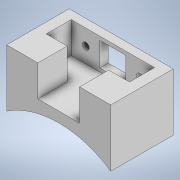
# Autodesk Inventor part: BracketForScope
Saved by Autodesk Inventor 2022.2 (Build 262287000, 287)
## iProperties
Created: 2021-12-26
Part Number: BracketForScope
Material: Generic
Document SubType Name: Modeling
Designer: robst
Density: 1 g/cm^3
Appearance: Default
Author: robst
Autodesk Inventor part; units mm, degrees
note: some values were not read from the file. Chosen so that the rebuilt part matches the saved one: direction of "Hole1".
ref_plane "YZ Plane" through (0, 0, 0) normal (1, 0, 0) x (0, 1, 0)
ref_plane "XZ Plane" through (0, 0, 0) normal (0, 1, 0) x (-1, 0, 0)
sketch "Sketch1" plane through (0, 0, 0) normal (0, 0, 1) x (1, 0, 0)
  arc A0 (25, 37.4166) -> (-25, 37.4166) centre (0, 0) ccw
  line L0 (0, 0) -> (0, 45) construction
  line L1 (0, 45) -> (25, 45)
  line L2 (0, 45) -> (-25, 45)
  line L3 (-25, 45) -> (-25, 37.4166)
  line L4 (25, 45) -> (25, 37.4166)
  line L5 (-25, 45) -> (25, 45)
  line L6 (25, 45) -> (25, 50)
  line L7 (25, 50) -> (-25, 50)
  line L8 (-25, 50) -> (-25, 45)
  dimension "d0" = 90
  dimension "d1" = 50
  dimension "d2" = 5
  constraints: 18 end point, 3 horizontal, 3 parallel, 3 point on circle, 2 vertical, 1 centre point, 1 coincident, 1 collinear, 1 perpendicular, 1 tangent
  measures "d0" diameter of A0
  measures "d1" distance of L1.end L2.end
  measures "d2" distance of L7.end L2.end
extrude "Extrusion1" add sketch "Sketch1" along normal mid plane 30
sketch "Sketch2" plane through (-25, 50, 15) normal (0, 1, 0) x (1, 0, 0)
  line L0 (50, 0) -> (0, 0) construction
  line L1 (25, 0) -> (25, 29.8898) construction
  line L2 (50, 0) -> (0, 0) construction
  line L3 (15, 0) -> (35, 0)
  line L4 (35, 0) -> (35, 14)
  line L5 (35, 14) -> (15, 14)
  line L6 (15, 14) -> (15, 0)
  line L7 (15, 0) -> (35, 14) construction
  line L8 (35, 0) -> (15, 14) construction
  line L9 (5, 14) -> (45, 14)
  line L10 (45, 14) -> (45, 26)
  line L11 (45, 26) -> (5, 26)
  line L12 (5, 26) -> (5, 14)
  line L13 (5, 14) -> (45, 26) construction
  line L14 (45, 14) -> (5, 26) construction
  line L15 (0, 30) -> (50, 30) projected
  line L16 (50, 30) -> (50, 0) projected
  line L17 (0, 0) -> (50, 0)
  line L18 (50, 0) -> (50, 30)
  line L19 (50, 30) -> (0, 30)
  line L20 (0, 30) -> (0, 0)
  point P0 (25, 15)
  point P1 (25, 7)
  point P2 (25, 20)
  point P3 (35, 14)
  point P4 (35, 0)
  point P5 (15, 0)
  point P6 (15, 14)
  dimension "d5" = 20
  dimension "d6" = 14
  dimension "d7" = 40
  dimension "d8" = 12
  dimension "d9" = 4
  dimension "d24" = 50
  constraints: 34 end point, 6 parallel, 5 midpoint, 5 perpendicular, 2 collinear, 2 point on line, 1 horizontal, 1 vertical
  measures "d5" distance of L4.end L5.end
  measures "d6" distance of L5.end L3.start
  measures "d7" distance of L10.end L11.end
  measures "d8" distance of L11.end L9.start
  measures "d9" distance between parallel lines of L11 L15
  measures "d24" distance between parallel lines of L18 L20
extrude "Extrusion2" add sketch "Sketch2" along normal blind 15 contours L17 L20 L15 L16 L4 L9 L10 L11 L12 L6
sketch "Sketch3" plane through (0, 0, -15) normal (0, 0, -1) x (-1, 0, 0)
  line L0 (-20, 50) -> (20, 50) projected
  line L1 (-25, 65) -> (25, 65) projected
  line L2 (20, 50) -> (20, 65) projected
  line L3 (-20, 50) -> (-20, 65) projected
  line L4 (0, 65) -> (0, 50) construction
  line L5 (20, 50) -> (20, 65) construction
  line L6 (20, 57.5) -> (-20, 57.5) construction
  line L7 (-6.25, 63.25) -> (-6.25, 51.75)
  line L8 (-6.25, 51.75) -> (6.25, 51.75)
  line L9 (6.25, 51.75) -> (6.25, 63.25)
  line L10 (6.25, 63.25) -> (-6.25, 63.25)
  line L11 (-6.25, 63.25) -> (6.25, 51.75) construction
  line L12 (-6.25, 51.75) -> (6.25, 63.25) construction
  point P0 (0, 0)
  point P1 (0, 57.5)
  dimension "d12" = 11.5
  dimension "d13" = 12.5
  constraints: 16 end point, 7 midpoint, 2 parallel, 1 perpendicular, 1 vertical
  measures "d12" distance of L8.end L9.end
  measures "d13" distance of L9.end L7.start
extrude "Extrusion3" cut sketch "Sketch3" against normal up to surface (4 mm away) contours L10 L9 L8 L7
sketch "Sketch5" plane through (0, 0, -15) normal (0, 0, -1) x (-1, 0, 0)
  line L0 (-20, 50) -> (20, 50) projected
  line L1 (20, 50) -> (20, 65) projected
  line L2 (-20, 50) -> (-20, 65) projected
  line L3 (-10, 50) -> (10, 50) construction
  line L4 (0, 50) -> (0, 65) construction
  line L5 (0, 57.5) -> (13, 57.5) construction
  line L6 (0, 57.5) -> (-13, 57.5) construction
  line L7 (6.25, 63.25) -> (6.25, 51.75) projected
  line L8 (-6.25, 51.75) -> (-6.25, 63.25) projected
  line L9 (6.25, 51.75) -> (6.25, 63.25) construction
  line L10 (6.25, 57.5) -> (-6.25, 57.5) construction
  line L11 (-6.25, 63.25) -> (-6.25, 51.75) construction
  point P0 (0, 0)
  dimension "d16" = 26
  constraints: 8 end point, 4 midpoint, 2 coincident, 2 collinear, 2 horizontal, 1 vertical
  measures "d16" distance of L5.end L6.end
hole "Hole1" at (13, 57.5, -15) at (-13, 57.5, -15) direction (0, 0, 1) diameter 3.264 end up to surface clearance for "Flat Head Machine Screw (82)" size "#4" standard "Ansi Unified Screw Threads"
ref_plane "Work Plane2" through (25, 37.4166, 0) normal (0, -1, 0) x (0, 0, 1)
sketch "Sketch6" plane through (25, 37.4166, 0) normal (0, -1, 0) x (0, 0, 1)
  line L0 (-15, 0) -> (-15, 50) projected
  line L1 (15, 50) -> (15, 0) projected
  line L2 (-15, 0) -> (15, 0) projected
  line L3 (-15, 50) -> (15, 50) projected
  line L4 (15, 0) -> (-15, 0) construction
  line L5 (0, 0) -> (0, 50) construction
  spline S0 degree 2 poles (0.1264, 5.3857) (0.1264, 4.8558) (-0.1507, 4.0681) (-0.4279, 3.7909) knots 0 0 0 1 2 2 2
  spline S1 degree 2 poles (-0.4279, 3.7909) (-0.7391, 3.4749) (-1.6143, 3.2172) (-2.2561, 3.2172) knots 0 0 0 1 2 2 2
  line L6 (-2.2561, 3.2172) -> (-6, 3.2172)
  line L7 (-6, 3.2172) -> (-6, 4.0146)
  line L8 (-6, 4.0146) -> (-2.2561, 4.0146)
  spline S2 degree 2 poles (-2.2561, 4.0146) (-1.8379, 4.0146) (-1.2739, 4.1216) (-1.0454, 4.2723) knots 0 0 0 1 2 2 2
  spline S3 degree 2 poles (-1.0454, 4.2723) (-0.8023, 4.4327) (-0.5543, 4.987) (-0.5543, 5.3857) knots 0 0 0 1 2 2 2
  spline S4 degree 2 poles (-0.5543, 5.3857) (-0.5543, 5.7601) (-0.8023, 6.3436) (-1.0454, 6.5041) knots 0 0 0 1 2 2 2
  spline S5 degree 2 poles (-1.0454, 6.5041) (-1.2739, 6.6548) (-1.8331, 6.7617) (-2.2366, 6.7617) knots 0 0 0 1 2 2 2
  line L9 (-2.2366, 6.7617) -> (-6, 6.7617)
  line L10 (-6, 6.7617) -> (-6, 7.5592)
  line L11 (-6, 7.5592) -> (-2.2561, 7.5592)
  spline S6 degree 2 poles (-2.2561, 7.5592) (-1.6288, 7.5592) (-0.7342, 7.3063) (-0.4279, 6.9854) knots 0 0 0 1 2 2 2
  spline S7 degree 2 poles (-0.4279, 6.9854) (-0.1459, 6.6985) (0.1264, 5.94) (0.1264, 5.3857) knots 0 0 0 1 2 2 2
  spline S8 degree 2 poles (0.107, 10.3744) (0.107, 9.7229) (-0.1653, 8.8088) (-0.3598, 8.4052) knots 0 0 0 1 2 2 2
  line L12 (-0.3598, 8.4052) -> (-1.3614, 8.4052)
  line L13 (-1.3614, 8.4052) -> (-1.3614, 8.4635)
  spline S9 degree 2 poles (-1.3614, 8.4635) (-0.9919, 8.8574) (-0.5835, 9.8541) (-0.5835, 10.316) knots 0 0 0 1 2 2 2
  spline S10 degree 2 poles (-0.5835, 10.316) (-0.5835, 10.9773) (-1.1329, 11.6532) (-1.5851, 11.6532) knots 0 0 0 1 2 2 2
  spline S11 degree 2 poles (-1.5851, 11.6532) (-1.9449, 11.6532) (-2.3922, 11.2982) (-2.5041, 10.9141) knots 0 0 0 1 2 2 2
  spline S12 degree 2 poles (-2.5041, 10.9141) (-2.5818, 10.637) (-2.6888, 10.175) (-2.7763, 9.8298) knots 0 0 0 1 2 2 2
  spline S13 degree 2 poles (-2.7763, 9.8298) (-2.859, 9.5186) (-3.107, 9.0276) (-3.3063, 8.8379) knots 0 0 0 1 2 2 2
  spline S14 degree 2 poles (-3.3063, 8.8379) (-3.5057, 8.6532) (-4.0405, 8.4489) (-4.3906, 8.4489) knots 0 0 0 1 2 2 2
  spline S15 degree 2 poles (-4.3906, 8.4489) (-5.1199, 8.4489) (-6.107, 9.5867) (-6.107, 10.4668) knots 0 0 0 1 2 2 2
  spline S16 degree 2 poles (-6.107, 10.4668) (-6.107, 10.9724) (-5.9076, 11.8671) (-5.718, 12.2512) knots 0 0 0 1 2 2 2
  line L14 (-5.718, 12.2512) -> (-4.765, 12.2512)
  line L15 (-4.765, 12.2512) -> (-4.765, 12.1929)
  spline S17 degree 2 poles (-4.765, 12.1929) (-5.0276, 11.906) (-5.4165, 11.0113) (-5.4165, 10.5203) knots 0 0 0 1 2 2 2
  spline S18 degree 2 poles (-5.4165, 10.5203) (-5.4165, 9.966) (-4.8963, 9.2804) (-4.4733, 9.2804) knots 0 0 0 1 2 2 2
  spline S19 degree 2 poles (-4.4733, 9.2804) (-4.094, 9.2804) (-3.6418, 9.684) (-3.5397, 10.0632) knots 0 0 0 1 2 2 2
  spline S20 degree 2 poles (-3.5397, 10.0632) (-3.4716, 10.316) (-3.2966, 11.0502) (-3.2237, 11.2934) knots 0 0 0 1 2 2 2
  spline S21 degree 2 poles (-3.2237, 11.2934) (-3.034, 11.9109) (-2.2707, 12.4846) (-1.7115, 12.4846) knots 0 0 0 1 2 2 2
  spline S22 degree 2 poles (-1.7115, 12.4846) (-1.3566, 12.4846) (-0.6759, 12.1977) (-0.4376, 11.94) knots 0 0 0 1 2 2 2
  spline S23 degree 2 poles (-0.4376, 11.94) (-0.175, 11.6532) (0.107, 10.9238) (0.107, 10.3744) knots 0 0 0 1 2 2 2
  spline S24 degree 2 poles (-1.8428, 17.3663) (-1.3955, 17.3663) (-0.7099, 17.0259) (-0.4862, 16.7439) knots 0 0 0 1 2 2 2
  spline S25 degree 2 poles (-0.4862, 16.7439) (-0.2237, 16.4036) (0, 15.6305) (0, 15.0178) knots 0 0 0 1 2 2 2
  line L16 (0, 15.0178) -> (0, 13.2966)
  line L17 (0, 13.2966) -> (-6, 13.2966)
  line L18 (-6, 13.2966) -> (-6, 14.8865)
  spline S26 degree 2 poles (-6, 14.8865) (-6, 15.5284) (-5.9173, 16.1702) (-5.7569, 16.4619) knots 0 0 0 1 2 2 2
  spline S27 degree 2 poles (-5.7569, 16.4619) (-5.5867, 16.7877) (-5.0276, 17.0843) (-4.6483, 17.0843) knots 0 0 0 1 2 2 2
  spline S28 degree 2 poles (-4.6483, 17.0843) (-4.2253, 17.0843) (-3.5543, 16.637) (-3.3647, 16.2431) knots 0 0 0 1 2 2 2
  line L19 (-3.3647, 16.2431) -> (-3.3355, 16.2431)
  spline S29 degree 2 poles (-3.3355, 16.2431) (-3.1896, 16.778) (-2.4165, 17.3663) (-1.8428, 17.3663) knots 0 0 0 1 2 2 2
  spline S30 degree 2 poles (-1.8088, 16.5348) (-2.1491, 16.5348) (-2.5867, 16.3404) (-2.7423, 16.0486) knots 0 0 0 1 2 2 2
  spline S31 degree 2 poles (-2.7423, 16.0486) (-2.8395, 15.859) (-2.8979, 15.4117) (-2.8979, 14.9984) knots 0 0 0 1 2 2 2
  line L20 (-2.8979, 14.9984) -> (-2.8979, 14.094)
  line L21 (-2.8979, 14.094) -> (-0.6807, 14.094)
  line L22 (-0.6807, 14.094) -> (-0.6807, 14.7407)
  spline S32 degree 2 poles (-0.6807, 14.7407) (-0.6807, 15.2658) (-0.778, 15.8687) (-0.9335, 16.1021) knots 0 0 0 1 2 2 2
  spline S33 degree 2 poles (-0.9335, 16.1021) (-1.094, 16.3258) (-1.4927, 16.5348) (-1.8088, 16.5348) knots 0 0 0 1 2 2 2
  spline S34 degree 2 poles (-4.5365, 16.2528) (-4.7504, 16.2528) (-5.0713, 16.107) (-5.1637, 15.9465) knots 0 0 0 1 2 2 2
  spline S35 degree 2 poles (-5.1637, 15.9465) (-5.2707, 15.752) (-5.3193, 15.2804) (-5.3193, 14.8574) knots 0 0 0 1 2 2 2
  line L23 (-5.3193, 14.8574) -> (-5.3193, 14.094)
  line L24 (-5.3193, 14.094) -> (-3.564, 14.094)
  line L25 (-3.564, 14.094) -> (-3.564, 14.9984)
  spline S36 degree 2 poles (-3.564, 14.9984) (-3.564, 15.3728) (-3.6418, 15.7277) (-3.7634, 15.9173) knots 0 0 0 1 2 2 2
  spline S37 degree 2 poles (-3.7634, 15.9173) (-3.8801, 16.1021) (-4.2545, 16.2528) (-4.5365, 16.2528) knots 0 0 0 1 2 2 2
  spline S38 degree 2 poles (-1.8428, 24.8055) (-1.3955, 24.8055) (-0.7099, 24.4652) (-0.4862, 24.1831) knots 0 0 0 1 2 2 2
  spline S39 degree 2 poles (-0.4862, 24.1831) (-0.2237, 23.8428) (0, 23.0697) (0, 22.4571) knots 0 0 0 1 2 2 2
  line L26 (0, 22.4571) -> (0, 20.7358)
  line L27 (0, 20.7358) -> (-6, 20.7358)
  line L28 (-6, 20.7358) -> (-6, 22.3258)
  spline S40 degree 2 poles (-6, 22.3258) (-6, 22.9676) (-5.9173, 23.6094) (-5.7569, 23.9011) knots 0 0 0 1 2 2 2
  spline S41 degree 2 poles (-5.7569, 23.9011) (-5.5867, 24.2269) (-5.0276, 24.5235) (-4.6483, 24.5235) knots 0 0 0 1 2 2 2
  spline S42 degree 2 poles (-4.6483, 24.5235) (-4.2253, 24.5235) (-3.5543, 24.0762) (-3.3647, 23.6823) knots 0 0 0 1 2 2 2
  line L29 (-3.3647, 23.6823) -> (-3.3355, 23.6823)
  spline S43 degree 2 poles (-3.3355, 23.6823) (-3.1896, 24.2172) (-2.4165, 24.8055) (-1.8428, 24.8055) knots 0 0 0 1 2 2 2
  spline S44 degree 2 poles (-1.8088, 23.9741) (-2.1491, 23.9741) (-2.5867, 23.7796) (-2.7423, 23.4878) knots 0 0 0 1 2 2 2
  spline S45 degree 2 poles (-2.7423, 23.4878) (-2.8395, 23.2982) (-2.8979, 22.8509) (-2.8979, 22.4376) knots 0 0 0 1 2 2 2
  line L30 (-2.8979, 22.4376) -> (-2.8979, 21.5332)
  line L31 (-2.8979, 21.5332) -> (-0.6807, 21.5332)
  line L32 (-0.6807, 21.5332) -> (-0.6807, 22.1799)
  spline S46 degree 2 poles (-0.6807, 22.1799) (-0.6807, 22.705) (-0.778, 23.3079) (-0.9335, 23.5413) knots 0 0 0 1 2 2 2
  spline S47 degree 2 poles (-0.9335, 23.5413) (-1.094, 23.765) (-1.4927, 23.9741) (-1.8088, 23.9741) knots 0 0 0 1 2 2 2
  spline S48 degree 2 poles (-4.5365, 23.6921) (-4.7504, 23.6921) (-5.0713, 23.5462) (-5.1637, 23.3857) knots 0 0 0 1 2 2 2
  spline S49 degree 2 poles (-5.1637, 23.3857) (-5.2707, 23.1912) (-5.3193, 22.7196) (-5.3193, 22.2966) knots 0 0 0 1 2 2 2
  line L33 (-5.3193, 22.2966) -> (-5.3193, 21.5332)
  line L34 (-5.3193, 21.5332) -> (-3.564, 21.5332)
  line L35 (-3.564, 21.5332) -> (-3.564, 22.4376)
  spline S50 degree 2 poles (-3.564, 22.4376) (-3.564, 22.812) (-3.6418, 23.1669) (-3.7634, 23.3566) knots 0 0 0 1 2 2 2
  spline S51 degree 2 poles (-3.7634, 23.3566) (-3.8801, 23.5413) (-4.2545, 23.6921) (-4.5365, 23.6921) knots 0 0 0 1 2 2 2
  line L36 (-3.6904, 27.9271) -> (-3.6904, 27.8882)
  spline S52 degree 2 poles (-3.6904, 27.8882) (-3.7147, 27.8006) (-3.7245, 27.611) (-3.7245, 27.4797) knots 0 0 0 1 2 2 2
  spline S53 degree 2 poles (-3.7245, 27.4797) (-3.7245, 27.1734) (-3.4571, 26.5705) (-3.1945, 26.2982) knots 0 0 0 1 2 2 2
  line L37 (-3.1945, 26.2982) -> (0, 26.2982)
  line L38 (0, 26.2982) -> (0, 25.5397)
  line L39 (0, 25.5397) -> (-4.5024, 25.5397)
  line L40 (-4.5024, 25.5397) -> (-4.5024, 26.2982)
  line L41 (-4.5024, 26.2982) -> (-3.8314, 26.2982)
  spline S54 degree 2 poles (-3.8314, 26.2982) (-4.201, 26.7115) (-4.5024, 27.329) (-4.5024, 27.6207) knots 0 0 0 1 2 2 2
  spline S55 degree 2 poles (-4.5024, 27.6207) (-4.5024, 27.7374) (-4.4927, 27.8541) (-4.4781, 27.9271) knots 0 0 0 1 2 2 2
  line L42 (-4.4781, 27.9271) -> (-3.6904, 27.9271)
  spline S56 degree 2 poles (-0.4765, 31.0243) (-0.4084, 30.9319) (-0.1653, 30.6207) (-0.0924, 30.4749) knots 0 0 0 1 2 2 2
  spline S57 degree 2 poles (-0.0924, 30.4749) (0.0146, 30.2755) (0.1264, 29.9011) (0.1264, 29.5608) knots 0 0 0 1 2 2 2
  spline S58 degree 2 poles (0.1264, 29.5608) (0.1264, 29.2836) (-0.0827, 28.7828) (-0.2723, 28.5932) knots 0 0 0 1 2 2 2
  spline S59 degree 2 poles (-0.2723, 28.5932) (-0.4571, 28.4133) (-1.0016, 28.1945) (-1.3031, 28.1945) knots 0 0 0 1 2 2 2
  spline S60 degree 2 poles (-1.3031, 28.1945) (-1.7699, 28.1945) (-2.4311, 28.5883) (-2.6207, 29.0162) knots 0 0 0 1 2 2 2
  spline S61 degree 2 poles (-2.6207, 29.0162) (-2.7958, 29.3955) (-2.9271, 30.4263) (-2.9611, 31.0243) knots 0 0 0 1 2 2 2
  line L43 (-2.9611, 31.0243) -> (-3.107, 31.0243)
  spline S62 degree 2 poles (-3.107, 31.0243) (-3.3695, 31.0243) (-3.6953, 30.8639) (-3.7877, 30.718) knots 0 0 0 1 2 2 2
  spline S63 degree 2 poles (-3.7877, 30.718) (-3.8801, 30.5721) (-3.9384, 30.154) (-3.9384, 29.9303) knots 0 0 0 1 2 2 2
  spline S64 degree 2 poles (-3.9384, 29.9303) (-3.9384, 29.6677) (-3.7828, 28.9579) (-3.6321, 28.6029) knots 0 0 0 1 2 2 2
  line L44 (-3.6321, 28.6029) -> (-3.6321, 28.5592)
  line L45 (-3.6321, 28.5592) -> (-4.4052, 28.5592)
  spline S65 degree 2 poles (-4.4052, 28.5592) (-4.4635, 28.7682) (-4.6094, 29.5511) (-4.6094, 29.9352) knots 0 0 0 1 2 2 2
  spline S66 degree 2 poles (-4.6094, 29.9352) (-4.6094, 30.4019) (-4.4635, 31.0389) (-4.2739, 31.2917) knots 0 0 0 1 2 2 2
  spline S67 degree 2 poles (-4.2739, 31.2917) (-4.0891, 31.5397) (-3.5008, 31.7828) (-3.0778, 31.7828) knots 0 0 0 1 2 2 2
  line L46 (-3.0778, 31.7828) -> (0, 31.7828)
  line L47 (0, 31.7828) -> (0, 31.0243)
  line L48 (0, 31.0243) -> (-0.4765, 31.0243)
  line L49 (-1.1086, 31.0243) -> (-2.3582, 31.0243)
  spline S68 degree 2 poles (-2.3582, 31.0243) (-2.3339, 30.752) (-2.2512, 29.9303) (-2.1734, 29.6726) knots 0 0 0 1 2 2 2
  spline S69 degree 2 poles (-2.1734, 29.6726) (-2.081, 29.3712) (-1.6969, 28.9773) (-1.3566, 28.9773) knots 0 0 0 1 2 2 2
  spline S70 degree 2 poles (-1.3566, 28.9773) (-0.9676, 28.9773) (-0.5737, 29.4149) (-0.5737, 29.8331) knots 0 0 0 1 2 2 2
  spline S71 degree 2 poles (-0.5737, 29.8331) (-0.5737, 30.188) (-0.8801, 30.7715) (-1.1086, 31.0243) knots 0 0 0 1 2 2 2
  spline S72 degree 2 poles (0.1021, 34.637) (0.1021, 34.1702) (-0.1848, 33.3971) (-0.4765, 33.1199) knots 0 0 0 1 2 2 2
  spline S73 degree 2 poles (-0.4765, 33.1199) (-0.7634, 32.8428) (-1.6483, 32.5365) (-2.2415, 32.5365) knots 0 0 0 1 2 2 2
  spline S74 degree 2 poles (-2.2415, 32.5365) (-2.8347, 32.5365) (-3.7002, 32.8525) (-3.9919, 33.1199) knots 0 0 0 1 2 2 2
  spline S75 degree 2 poles (-3.9919, 33.1199) (-4.2885, 33.3874) (-4.6045, 34.1799) (-4.6045, 34.637) knots 0 0 0 1 2 2 2
  spline S76 degree 2 poles (-4.6045, 34.637) (-4.6045, 35.0065) (-4.3955, 35.6969) (-4.2593, 35.9643) knots 0 0 0 1 2 2 2
  line L50 (-4.2593, 35.9643) -> (-3.4084, 35.9643)
  line L51 (-3.4084, 35.9643) -> (-3.4084, 35.9206)
  spline S77 degree 2 poles (-3.4084, 35.9206) (-3.4765, 35.8379) (-3.6515, 35.5851) (-3.7439, 35.4052) knots 0 0 0 1 2 2 2
  spline S78 degree 2 poles (-3.7439, 35.4052) (-3.8217, 35.2447) (-3.9433, 34.8169) (-3.9433, 34.6224) knots 0 0 0 1 2 2 2
  spline S79 degree 2 poles (-3.9433, 34.6224) (-3.9433, 34.034) (-3.0535, 33.3193) (-2.2415, 33.3193) knots 0 0 0 1 2 2 2
  spline S80 degree 2 poles (-2.2415, 33.3193) (-1.4489, 33.3193) (-0.5592, 34.0097) (-0.5592, 34.6224) knots 0 0 0 1 2 2 2
  spline S81 degree 2 poles (-0.5592, 34.6224) (-0.5592, 34.9919) (-0.8655, 35.6629) (-1.1037, 35.9206) knots 0 0 0 1 2 2 2
  line L52 (-1.1037, 35.9206) -> (-1.1037, 35.9643)
  line L53 (-1.1037, 35.9643) -> (-0.2528, 35.9643)
  spline S82 degree 2 poles (-0.2528, 35.9643) (-0.1994, 35.8525) (-0.0486, 35.5122) (-0.0146, 35.376) knots 0 0 0 1 2 2 2
  spline S83 degree 2 poles (-0.0146, 35.376) (0.0438, 35.1815) (0.1021, 34.8752) (0.1021, 34.637) knots 0 0 0 1 2 2 2
  line L54 (0, 40.3841) -> (0, 39.3874)
  line L55 (0, 39.3874) -> (-2.1734, 37.7148)
  line L56 (-2.1734, 37.7148) -> (-1.8817, 37.4133)
  line L57 (-1.8817, 37.4133) -> (0, 37.4133)
  line L58 (0, 37.4133) -> (0, 36.6548)
  line L59 (0, 36.6548) -> (-6.2674, 36.6548)
  line L60 (-6.2674, 36.6548) -> (-6.2674, 37.4133)
  line L61 (-6.2674, 37.4133) -> (-2.6013, 37.4133)
  line L62 (-2.6013, 37.4133) -> (-4.5024, 39.1929)
  line L63 (-4.5024, 39.1929) -> (-4.5024, 40.1361)
  line L64 (-4.5024, 40.1361) -> (-2.6207, 38.2885)
  line L65 (-2.6207, 38.2885) -> (0, 40.3841)
  spline S84 degree 2 poles (0.1021, 42.718) (0.1021, 41.6386) (-1.1086, 40.4522) (-2.2269, 40.4522) knots 0 0 0 1 2 2 2
  spline S85 degree 2 poles (-2.2269, 40.4522) (-3.3258, 40.4522) (-4.6288, 41.6045) (-4.6288, 42.5332) knots 0 0 0 1 2 2 2
  spline S86 degree 2 poles (-4.6288, 42.5332) (-4.6288, 42.9514) (-4.3857, 43.5981) (-4.128, 43.8363) knots 0 0 0 1 2 2 2
  spline S87 degree 2 poles (-4.128, 43.8363) (-3.8703, 44.0794) (-3.1264, 44.3371) (-2.5867, 44.3371) knots 0 0 0 1 2 2 2
  line L66 (-2.5867, 44.3371) -> (-2.1734, 44.3371)
  line L67 (-2.1734, 44.3371) -> (-2.1734, 41.2204)
  spline S88 degree 2 poles (-2.1734, 41.2204) (-1.3906, 41.2204) (-0.5592, 42.0081) (-0.5592, 42.7083) knots 0 0 0 1 2 2 2
  spline S89 degree 2 poles (-0.5592, 42.7083) (-0.5592, 42.9562) (-0.671, 43.4376) (-0.7585, 43.6321) knots 0 0 0 1 2 2 2
  spline S90 degree 2 poles (-0.7585, 43.6321) (-0.8558, 43.8363) (-1.0259, 44.1183) (-1.1037, 44.2107) knots 0 0 0 1 2 2 2
  line L68 (-1.1037, 44.2107) -> (-1.1037, 44.2545)
  line L69 (-1.1037, 44.2545) -> (-0.2771, 44.2545)
  spline S91 degree 2 poles (-0.2771, 44.2545) (-0.2237, 44.1232) (-0.0681, 43.7245) (-0.0243, 43.5689) knots 0 0 0 1 2 2 2
  spline S92 degree 2 poles (-0.0243, 43.5689) (0.0389, 43.3501) (0.1021, 42.9903) (0.1021, 42.718) knots 0 0 0 1 2 2 2
  spline S93 degree 2 poles (-2.752, 43.5981) (-3.0583, 43.5883) (-3.5057, 43.4619) (-3.6564, 43.3404) knots 0 0 0 1 2 2 2
  spline S94 degree 2 poles (-3.6564, 43.3404) (-3.8266, 43.2091) (-4.0065, 42.7958) (-4.0065, 42.4895) knots 0 0 0 1 2 2 2
  spline S95 degree 2 poles (-4.0065, 42.4895) (-4.0065, 42.188) (-3.8266, 41.765) (-3.6515, 41.59) knots 0 0 0 1 2 2 2
  spline S96 degree 2 poles (-3.6515, 41.59) (-3.4716, 41.4198) (-3.0389, 41.2447) (-2.752, 41.2204) knots 0 0 0 1 2 2 2
  line L70 (-2.752, 41.2204) -> (-2.752, 43.5981)
  spline S97 degree 2 poles (0.0875, 46.4668) (0.0875, 45.8493) (-0.6175, 45.154) (-1.3809, 45.154) knots 0 0 0 1 2 2 2
  line L71 (-1.3809, 45.154) -> (-3.8752, 45.154)
  line L72 (-3.8752, 45.154) -> (-3.8752, 44.6434)
  line L73 (-3.8752, 44.6434) -> (-4.5024, 44.6434)
  line L74 (-4.5024, 44.6434) -> (-4.5024, 45.154)
  line L75 (-4.5024, 45.154) -> (-5.7958, 45.154)
  line L76 (-5.7958, 45.154) -> (-5.7958, 45.9125)
  line L77 (-5.7958, 45.9125) -> (-4.5024, 45.9125)
  line L78 (-4.5024, 45.9125) -> (-4.5024, 47.3079)
  line L79 (-4.5024, 47.3079) -> (-3.8752, 47.3079)
  line L80 (-3.8752, 47.3079) -> (-3.8752, 45.9125)
  line L81 (-3.8752, 45.9125) -> (-1.731, 45.9125)
  spline S98 degree 2 poles (-1.731, 45.9125) (-1.3906, 45.9125) (-1.0162, 45.9368) (-0.8558, 46.0195) knots 0 0 0 1 2 2 2
  spline S99 degree 2 poles (-0.8558, 46.0195) (-0.7147, 46.0875) (-0.5737, 46.3938) (-0.5737, 46.6564) knots 0 0 0 1 2 2 2
  spline S100 degree 2 poles (-0.5737, 46.6564) (-0.5737, 46.8412) (-0.6856, 47.1864) (-0.7196, 47.2642) knots 0 0 0 1 2 2 2
  line L82 (-0.7196, 47.2642) -> (-0.7196, 47.3079)
  line L83 (-0.7196, 47.3079) -> (-0.0389, 47.3079)
  spline S101 degree 2 poles (-0.0389, 47.3079) (0.0194, 47.094) (0.0875, 46.6564) (0.0875, 46.4668) knots 0 0 0 1 2 2 2
  spline S102 degree 2 poles (5.7169, 20.1596) (6.1059, 20.1596) (6.806, 19.8825) (7.0492, 19.6345) knots 0 0 0 1 2 2 2
  spline S103 degree 2 poles (7.0492, 19.6345) (7.3555, 19.3233) (7.6715, 18.4822) (7.6715, 17.8404) knots 0 0 0 1 2 2 2
  line L84 (7.6715, 17.8404) -> (7.6715, 17.1645)
  line L85 (7.6715, 17.1645) -> (9.9082, 17.1645)
  line L86 (9.9082, 17.1645) -> (9.9082, 16.3671)
  line L87 (9.9082, 16.3671) -> (3.9082, 16.3671)
  line L88 (3.9082, 16.3671) -> (3.9082, 17.8744)
  spline S104 degree 2 poles (3.9082, 17.8744) (3.9082, 18.4092) (4.0832, 19.158) (4.2825, 19.4449) knots 0 0 0 1 2 2 2
  spline S105 degree 2 poles (4.2825, 19.4449) (4.5111, 19.7804) (5.2161, 20.1596) (5.7169, 20.1596) knots 0 0 0 1 2 2 2
  spline S106 degree 2 poles (5.7412, 19.3282) (5.43, 19.3282) (4.973, 19.1143) (4.8271, 18.8955) knots 0 0 0 1 2 2 2
  spline S107 degree 2 poles (4.8271, 18.8955) (4.7007, 18.7058) (4.5986, 18.2002) (4.5986, 17.8258) knots 0 0 0 1 2 2 2
  line L89 (4.5986, 17.8258) -> (4.5986, 17.1645)
  line L90 (4.5986, 17.1645) -> (6.9908, 17.1645)
  line L91 (6.9908, 17.1645) -> (6.9908, 17.7091)
  spline S108 degree 2 poles (6.9908, 17.7091) (6.9908, 18.1953) (6.8352, 18.7934) (6.631, 18.9878) knots 0 0 0 1 2 2 2
  spline S109 degree 2 poles (6.631, 18.9878) (6.4511, 19.1677) (6.0281, 19.3282) (5.7412, 19.3282) knots 0 0 0 1 2 2 2
  line L92 (3.9082, 25.2699) -> (9.9082, 23.2034)
  line L93 (9.9082, 23.2034) -> (9.9082, 22.3428)
  line L94 (9.9082, 22.3428) -> (3.9082, 20.2763)
  line L95 (3.9082, 20.2763) -> (3.9082, 21.1321)
  line L96 (3.9082, 21.1321) -> (8.8919, 22.795)
  line L97 (8.8919, 22.795) -> (3.9082, 24.4579)
  line L98 (3.9082, 24.4579) -> (3.9082, 25.2699)
  spline S110 degree 2 poles (6.9082, 29.4757) (8.5224, 29.4757) (10.0346, 28.5373) (10.0346, 27.56) knots 0 0 0 1 2 2 2
  spline S111 degree 2 poles (10.0346, 27.56) (10.0346, 26.5681) (8.4932, 25.6394) (6.913, 25.6394) knots 0 0 0 1 2 2 2
  spline S112 degree 2 poles (6.913, 25.6394) (5.289, 25.6394) (3.7866, 26.5778) (3.7866, 27.56) knots 0 0 0 1 2 2 2
  spline S113 degree 2 poles (3.7866, 27.56) (3.7866, 28.547) (5.3425, 29.4757) (6.9082, 29.4757) knots 0 0 0 1 2 2 2
  spline S114 degree 2 poles (8.7364, 28.4449) (8.4398, 28.5616) (7.5257, 28.6588) (6.9082, 28.6588) knots 0 0 0 1 2 2 2
  spline S115 degree 2 poles (6.9082, 28.6588) (6.2907, 28.6588) (5.3814, 28.5616) (5.0751, 28.44) knots 0 0 0 1 2 2 2
  spline S116 degree 2 poles (5.0751, 28.44) (4.7688, 28.3185) (4.4527, 27.8955) (4.4527, 27.56) knots 0 0 0 1 2 2 2
  spline S117 degree 2 poles (4.4527, 27.56) (4.4527, 27.2245) (4.7688, 26.7917) (5.0848, 26.6653) knots 0 0 0 1 2 2 2
  spline S118 degree 2 poles (5.0848, 26.6653) (5.3911, 26.5438) (6.3247, 26.4562) (6.913, 26.4562) knots 0 0 0 1 2 2 2
  spline S119 degree 2 poles (6.913, 26.4562) (7.5451, 26.4562) (8.3911, 26.534) (8.7218, 26.6605) knots 0 0 0 1 2 2 2
  spline S120 degree 2 poles (8.7218, 26.6605) (9.033, 26.7771) (9.3684, 27.2099) (9.3684, 27.56) knots 0 0 0 1 2 2 2
  spline S121 degree 2 poles (9.3684, 27.56) (9.3684, 27.8906) (9.0524, 28.3233) (8.7364, 28.4449) knots 0 0 0 1 2 2 2
  line L99 (9.9082, 33.9441) -> (9.9082, 30.2439)
  line L100 (9.9082, 30.2439) -> (9.0573, 30.2439)
  spline S122 degree 2 poles (9.0573, 30.2439) (8.6829, 30.6426) (7.9876, 31.3525) (7.6132, 31.6929) knots 0 0 0 1 2 2 2
  spline S123 degree 2 poles (7.6132, 31.6929) (6.8595, 32.3784) (5.9552, 32.8793) (5.4738, 32.8793) knots 0 0 0 1 2 2 2
  spline S124 degree 2 poles (5.4738, 32.8793) (5.221, 32.8793) (4.8417, 32.7237) (4.7201, 32.5827) knots 0 0 0 1 2 2 2
  spline S125 degree 2 poles (4.7201, 32.5827) (4.5986, 32.4417) (4.477, 32.0721) (4.477, 31.8485) knots 0 0 0 1 2 2 2
  spline S126 degree 2 poles (4.477, 31.8485) (4.477, 31.6345) (4.584, 31.1969) (4.6667, 30.9976) knots 0 0 0 1 2 2 2
  spline S127 degree 2 poles (4.6667, 30.9976) (4.7347, 30.8274) (4.9292, 30.5113) (4.9973, 30.4141) knots 0 0 0 1 2 2 2
  line L101 (4.9973, 30.4141) -> (4.9973, 30.3703)
  line L102 (4.9973, 30.3703) -> (4.1415, 30.3703)
  spline S128 degree 2 poles (4.1415, 30.3703) (4.02, 30.6183) (3.7817, 31.5081) (3.7817, 31.9068) knots 0 0 0 1 2 2 2
  spline S129 degree 2 poles (3.7817, 31.9068) (3.7817, 32.748) (4.6715, 33.6961) (5.43, 33.6961) knots 0 0 0 1 2 2 2
  spline S130 degree 2 poles (5.43, 33.6961) (5.785, 33.6961) (6.3782, 33.5308) (6.631, 33.3849) knots 0 0 0 1 2 2 2
  spline S131 degree 2 poles (6.631, 33.3849) (6.8936, 33.2391) (7.409, 32.816) (7.6569, 32.5827) knots 0 0 0 1 2 2 2
  spline S132 degree 2 poles (7.6569, 32.5827) (8.0702, 32.2034) (8.9552, 31.2747) (9.2129, 30.9976) knots 0 0 0 1 2 2 2
  line L103 (9.2129, 30.9976) -> (9.2129, 33.9441)
  line L104 (9.2129, 33.9441) -> (9.9082, 33.9441)
  point P0 (0, 25)
  constraints: 2 end point, 2 midpoint, 1 vertical
emboss "Emboss1" sketch "Sketch6" operation cut depth 1 direction (0, -1, 0) wrap yes faces at (14.4644, 42.612, 5) contours S0 S1 L6 L7 L8 S2 S3 S4 S5 L9 L10 L11 S6 S7 | S8 L12 L13 S9 S10 S11 S12 S13 S14 S15 S16 L14 L15 S17 S18 S19 S20 S21 S22 S23 | S24 S25 L16 L17 L18 S26 S27 S28 L19 S29 | S38 S39 L26 L27 L28 S40 S41 S42 L29 S43 | L36 S52 S53 L37 L38 L39 L40 L41 S54 S55 L42 | S56 S57 S58 S59 S60 S61 L43 S62 S63 S64 L44 L45 S65 S66 S67 L46 L47 L48 | S72 S73 S74 S75 S76 L50 L51 S77 S78 S79 S80 S81 L52 L53 S82 S83 | L54 L55 L56 L57 L58 L59 L60 L61 L62 L63 L64 L65 | S84 S85 S86 S87 L66 L67 S88 S89 S90 L68 L69 S91 S92 | S97 L71 L72 L73 L74 L75 L76 L77 L78 L79 L80 L81 S98 S99 S100 L82 L83 S101 | S102 S103 L84 L85 L86 L87 L88 S104 S105 | L92 L93 L94 L95 L96 L97 L98 | S110 S111 S112 S113 | L99 L100 S122 S123 S124 S125 S126 S127 L101 L102 S128 S129 S130 S131 S132 L103 L104
equation "\"d0\" = baseDiameter"
equation "\"d1\" = outerWidth"
equation "\"baseDiameter\" = 90"
equation "\"wallThickness\" = 4"
equation "\"outerWidth\" = 50"
body "Solid1"
